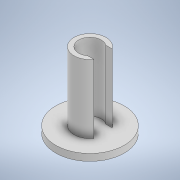
# Autodesk Inventor part: fsrBase
Saved by Autodesk Inventor 2022 (Build 260153000, 153)
## iProperties
Created: 2021-10-23
Part Number: fsrBase
Material: Generic
Document SubType Name: Modeling
Designer: liwei
Density: 1 g/cm^3
Appearance: Default
Author: liwei
Autodesk Inventor part; units mm, degrees
ref_plane "YZ Plane" through (0, 0, 0) normal (1, 0, 0) x (0, 1, 0)
ref_plane "XZ Plane" through (0, 0, 0) normal (0, 1, 0) x (-1, 0, 0)
ref_plane "XY Plane" through (0, 0, 0) normal (0, 0, 1) x (1, 0, 0)
sketch "Sketch1" plane through (0, 0, 0) normal (0, 1, 0) x (-1, 0, 0)
  point P0 (0, 0)
sketch "Sketch2" plane through (0, 0, 0) normal (0, 1, 0) x (-1, 0, 0)
  circle A0 centre (0, 0) radius 5
  circle A1 centre (0, 0) radius 7
  line L0 (-0.0083, 4) -> (-10.0083, 4)
  line L1 (-10.0083, 4) -> (-10.0083, -4)
  line L2 (-10.0083, -4) -> (-0.0083, -4)
  line L3 (-0.0083, -4) -> (-0.0083, 4)
  point P0 (-3, -4)
  point P1 (-5.7446, -4)
  point P2 (-5.7446, 4)
  point P3 (-3, 4)
  dimension "d0" = 10
  dimension "d1" = 14
  dimension "d2" = 10
  dimension "d3" = 8
  dimension "d4" = 3
  constraints: 8 end point, 2 centre point, 2 coincident, 2 parallel, 1 horizontal, 1 perpendicular
  measures "d0" diameter of A0
  measures "d1" diameter of A1
  measures "d2" distance of L2.end L1.end
  measures "d3" distance of L0.end L1.end
  measures "d4" distance edge to line of A1 L2
extrude "Extrusion1" add sketch "Sketch2" along normal blind 30 contours A0 L0 A1 L2 picked at (-4.4748, -4.4019)
sketch "Sketch3" plane through (0, 0, 0) normal (0, -1, 0) x (1, 0, 0)
  circle A0 centre (0, 0) radius 15
  dimension "d7" = 30
  constraints: 1 centre point, 1 coincident
  measures "d7" diameter of A0
extrude "Extrusion2" add sketch "Sketch3" along normal blind 3
body "Solid1"
